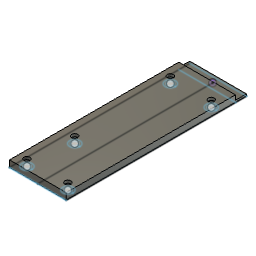
MB-RL7021-11-M5StickC Bottom v4 (Autodesk Fusion 360 design; units mm, degrees)
Autodesk Fusion 360 part; units mm, degrees
sketch "スケッチ1" plane through (0, 0, 0) normal (0, 1, 0) x (1, 0, 0)
  line L0 (-10.375, 2) -> (10.375, 2)
  line L1 (10.375, 2) -> (10.375, -64)
  line L2 (10.375, -64) -> (-10.375, -64)
  line L3 (-10.375, -64) -> (-10.375, 2)
  line L4 (0, 0) -> (0, -64)
  circle A0 centre (7.5, -8) radius 1.1
  circle A1 centre (7.5, -8) radius 1.85
  circle A2 centre (7.5, -60.5) radius 1.1
  circle A3 centre (7.5, -60.5) radius 1.85
  line L5 (-10.375, -2) -> (10.375, -2)
  circle A4 centre (-7.5, -8) radius 1.85
  circle A5 centre (-7.5, -8) radius 1.1
  circle A6 centre (-7.5, -60.5) radius 1.85
  circle A7 centre (-7.5, -60.5) radius 1.1
  circle A8 centre (-6, -44.5) radius 1.1
  circle A9 centre (-6, -44.5) radius 1.85
  dimension "d1" = 66
  dimension "d2" = 20.75
  dimension "d3" = 10.375
  dimension "d4" = 2.2
  dimension "d6" = 10
  dimension "d7" = 3.7
  dimension "d8" = 2.2
  dimension "d9" = 3.7
  dimension "d11" = 62.5
  dimension "d12" = 7.5
  dimension "d13" = 7.5
  dimension "d14" = 4
  dimension "d27" = 3.7
  dimension "d28" = 2.2
  dimension "d29" = 6
  dimension "d30" = 46.5
  constraint horizontal L0
  constraint vertical L1
  constraint horizontal L2
  constraint vertical L3
  constraint coincident L4.start origin
  constraint coincident L2 L4.end
  constraint perpendicular L2 L4
  constraint concentric A0 A1
  constraint concentric A2 A3
  constraint coincident L3 L5.start
  constraint coincident L1 L5.end
  constraint perpendicular L1 L5
  constraint symmetric L4 A0 A5
  constraint symmetric L4 A1 A4
  constraint symmetric L4 A2 A7
  constraint symmetric L4 A3 A6
  constraint concentric A8 A9
  measures "d1" distance of L0.start L2.end
  measures "d2" distance of L0.start L0.end
  measures "d3" distance of L3 L4
  measures "d4" diameter of A0
  measures "d6" distance of L0 A0.centre
  measures "d7" diameter of A1
  measures "d8" diameter of A2
  measures "d9" diameter of A3
  measures "d11" distance of L0 A2.centre
  measures "d12" distance of L4 A2.centre
  measures "d13" distance of L4 A0.centre
  measures "d14" distance of L0 L5
  measures "d27" diameter of A9
  measures "d28" diameter of A8
  measures "d29" distance of L4 A8.centre
  measures "d30" distance of L0 A8.centre
extrude "押し出し4" add sketch "スケッチ1" along normal blind 0.7 contours L0 L1 L3 L5 | L2 L3 L4 L5 | L1 L2 L4 L5 | A1 | A3 | A4 | A6 | A8 | A9 makes body 1
extrude "押し出し5" add sketch "スケッチ1" along normal blind 2.4 separate body contours L2 L3 L4 L5 | L1 L2 L4 L5 | A1 | A3 | A4 | A6 | A8 | A9 makes body 2
combine "結合1" operation add target body 2 tool bodies 1
extrude "押し出し6" cut sketch "スケッチ1" along normal blind 1.4 contours A1 | A3 | A4 | A6 bodies 2
extrude "押し出し7" cut sketch "スケッチ1" along normal blind 2.4 contours A8 bodies 2
extrude "押し出し8" cut sketch "スケッチ1" along normal blind 1.4 contours A9 bodies 2
